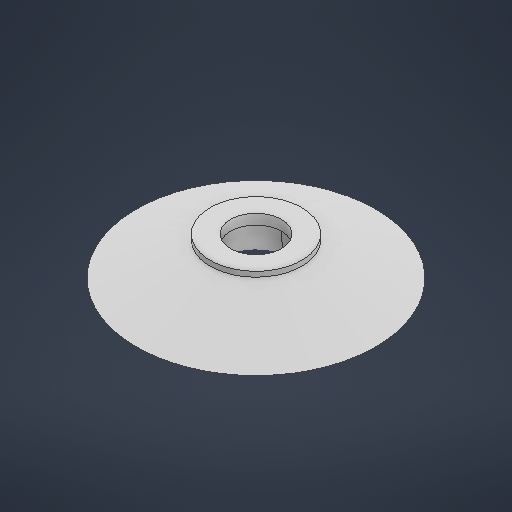
# Autodesk Inventor part: Статор диска
Saved by Autodesk Inventor 2026 (Build 300175000, 175)
## iProperties
Created: 2025-08-13
Part Number: Статор диска
Material: Типовые
Document SubType Name: Modeling
Designer: kvm13
Density: 1 g/cm^3
Appearance: По умолчанию
Author: kvm13
Autodesk Inventor part; units mm, degrees
ref_plane "YZ Plane" through (0, 0, 0) normal (1, 0, 0) x (0, 1, 0)
ref_plane "XZ Plane" through (0, 0, 0) normal (0, 1, 0) x (-1, 0, 0)
ref_plane "XY Plane" through (0, 0, 0) normal (0, 0, 1) x (1, 0, 0)
sketch "Эскиз1" plane through (0, 0, 0) normal (1, 0, 0) x (0, 1, 0)
  line L0 (6.0175, 5.2485) -> (7.0348, 5.2485)
  line L1 (0.5348, 2.7485) -> (0.5348, -15.7515)
  line L2 (0.5348, 2.7485) -> (0.5348, 2.7485)
  line L3 (0.5348, 2.7485) -> (0.5348, 5.2485) construction
  line L4 (0.5348, 5.2485) -> (6.0175, 5.2485) construction
  spline S0 degree 2 poles (0.5348, 2.7485) (0.5348, 5.2485) (6.0175, 5.2485) knots 1 1 1 2 2 2
  line L5 (3.5175, 7.7485) -> (4.5348, 7.7485)
  line L6 (-1.9652, 5.2485) -> (-1.9652, -13.2515)
  line L7 (-1.9652, 5.2485) -> (-1.9652, 5.2485)
  line L8 (-1.9652, 5.2485) -> (-1.9652, 7.7485) construction
  spline S1 degree 2 poles (-1.9652, 5.2485) (-1.9652, 7.7485) (3.5175, 7.7485) knots 1 1 1 2 2 2
  line L9 (-1.9652, 7.7485) -> (3.5175, 7.7485) construction
  line L10 (4.5348, 7.7485) -> (4.5348, 10.2485)
  line L11 (-1.9652, -13.2515) -> (3.8563, -13.2515)
  line L12 (7.0348, 5.2485) -> (7.0348, 1.2485)
  line L13 (7.0348, 1.2485) -> (0.5348, -13.2515)
  line L14 (7.0348, 5.2485) -> (8.0348, 5.2485)
  line L15 (8.0348, 5.2485) -> (8.0348, 1.2485)
  line L16 (8.0348, 1.2485) -> (7.0348, 1.2485)
  line L17 (7.0348, 10.2485) -> (0.2011, 10.2485)
  point P0 (0, 0)
  point P1 (1.5611, 5.7302)
  dimension "d4" = 2.5
  dimension "d5" = 2.5
  dimension "d6" = 2.5
  dimension "d7" = 4
  dimension "d8" = 1
  constraints: 28 end point, 6 vertical, 3 horizontal, 2 perpendicular, 2 point on line, 6 other
  measures "d4" horizontal distance of L0.end L5.end
  measures "d5" distance of L5.end L10.end
  measures "d6" horizontal distance of L0.end L5.end
  measures "d7" distance of L0.end L12.end
  measures "d8" distance of L0.end L14.end
revolve "Вращение1" add sketch "Эскиз1" angle 360 about axis through (0, 7.0348, 10.2485) along (0, -1, 0)
